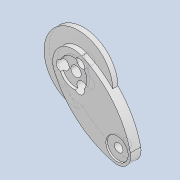
# Autodesk Inventor part: 原動節4
Saved by Autodesk Inventor 2020 (Build 240168000, 168)
## iProperties
Created: 2020-10-27
Part Number: 原動節4
Material: アルミニウム 2014-T4
Document SubType Name: Modeling
Designer: AA19065
Density: 2.8 g/cm^3
Appearance: サテン
Mass: 2.64814 g
Surface Area: 11.2941 cm^2
Volume: 0.945763 cm^3
Author: AA19065
Autodesk Inventor part; units mm, degrees
ref_plane "YZ Plane" through (0, 0, 0) normal (1, 0, 0) x (0, 1, 0)
ref_plane "XZ Plane" through (0, 0, 0) normal (0, 1, 0) x (-1, 0, 0)
ref_plane "XY Plane" through (0, 0, 0) normal (0, 0, 1) x (1, 0, 0)
sketch "スケッチ1" plane through (0, 0, 0) normal (0, 0, 1) x (1, 0, 0)
  circle A0 centre (-10.9779, 15.759) radius 1.5
  circle A1 centre (-12.7279, 12.7279) radius 1.25
  circle A2 centre (-16.2279, 12.7279) radius 1.5
  circle A3 centre (-10.9779, 9.6968) radius 1.5
  circle A4 centre (-12.7279, 12.7279) radius 6
  circle A5 centre (0, 0) radius 4
  circle A6 centre (0, 0) radius 1.25
  arc A7 (3.9022, 0.8792) -> (-10.2779, 18.2049) centre (-20.4864, -4.6158) ccw
  arc A8 (-18.2049, 10.2779) -> (-0.8792, -3.9022) centre (4.6158, 20.4864) ccw
  circle A9 centre (-12.7279, 12.7279) radius 1.5
  circle A10 centre (-16.2279, 12.7279) radius 1.5
  circle A11 centre (-12.7279, 12.7279) radius 1.25
  circle A12 centre (-10.9779, 9.6968) radius 1.5
  circle A13 centre (-10.9779, 15.759) radius 1.5
  circle A14 centre (-12.7279, 12.7279) radius 6
  circle A15 centre (0, 0) radius 4
  circle A16 centre (0, 0) radius 1.25
  arc A17 (3.9022, 0.8792) -> (-10.2779, 18.2049) centre (-20.4864, -4.6158) ccw
  arc A18 (-18.2049, 10.2779) -> (-0.8792, -3.9022) centre (4.6158, 20.4864) ccw
  circle A19 centre (-12.7279, 12.7279) radius 1.5
  dimension "d0" = 8
  dimension "d1" = 2.5
  dimension "d2" = 25
  dimension "d3" = 3
  dimension "d6" = 8
  dimension "d7" = 2.5
  dimension "d8" = 25
  dimension "d9" = 3
  dimension "d19" = 3
  dimension "d20" = 2.5
  constraints: 20 centre point, 16 point on circle, 9 equal radius, 8 tangent, 7 coincident, 5 concentric, 5 other
  measures "d0" diameter of A5
  measures "d1" diameter of A6
  measures "d2" radius of A7
  measures "d3" diameter of A9
  measures "d6" diameter of A15
  measures "d7" diameter of A16
  measures "d8" radius of A17
  measures "d9" diameter of A19
  measures "d19" diameter of A0
  measures "d20" diameter of A11
extrude "押し出し1" add sketch "スケッチ1" along normal blind 3 contours A4 | A4 A7 A5 A8 | A5
sketch "スケッチ2" plane through (0, 0, 3) normal (0, 0, 1) x (1, 0, 0)
  circle A0 centre (-12.7279, 12.7279) radius 1.5 projected
  circle A1 centre (-12.7279, 12.7279) radius 4
  point P0 (0, 0)
  dimension "d10" = 8
  constraints: 1 centre point, 1 coincident
  measures "d10" diameter of A1
extrude "押し出し2" cut sketch "スケッチ2" against normal blind 0.8
sketch "スケッチ3" plane through (0, 0, 0) normal (0, 0, -1) x (-1, 0, 0)
  circle A0 centre (12.7279, 12.7279) radius 1.5 projected
  circle A1 centre (12.7279, 12.7279) radius 10
  arc A2 (0.8792, -3.9022) -> (18.2049, 10.2779) centre (-4.6158, 20.4864) ccw projected
  arc A3 (18.2049, 10.2779) -> (10.2779, 18.2049) centre (12.7279, 12.7279) ccw projected
  arc A4 (10.2779, 18.2049) -> (-3.9022, 0.8792) centre (20.4864, -4.6158) ccw projected
  arc A5 (-3.9022, 0.8792) -> (0.8792, -3.9022) centre (0, 0) ccw projected
  circle A6 centre (0, 0) radius 1.25 projected
  circle A7 centre (16.2279, 12.7279) radius 1.5 projected
  circle A8 centre (12.7279, 12.7279) radius 1.5 projected
  circle A9 centre (10.9779, 9.6968) radius 1.5 projected
  circle A10 centre (10.9779, 15.759) radius 1.5 projected
  point P0 (12.9839, 2.7312)
  point P1 (2.7312, 12.9839)
  dimension "d13" = 20
  constraints: 1 centre point, 1 coincident
  measures "d13" diameter of A1
extrude "押し出し3" add sketch "スケッチ3" against normal blind 1.5 contours A1 A2 A3 A4 picked at (8.342, 18.6804)
sketch "スケッチ4" plane through (0, 0, 3) normal (0, 0, 1) x (1, 0, 0)
  circle A0 centre (0, 0) radius 3.25
  dimension "d16" = 6.5
  constraints: 1 centre point, 1 coincident
  measures "d16" diameter of A0
extrude "押し出し4" cut sketch "スケッチ4" against normal blind 0.5
equation "\"d1\" = d20"
equation "\"d3\" = d9"
equation "\"d7\" = d1"
equation "\"d9\" = d19"
